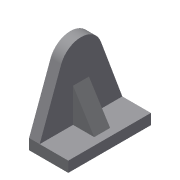
# Autodesk Inventor part: Bracket
Saved by Autodesk Inventor 2022 (Build 260148000, 148)
## iProperties
Created: 2007-03-01
Part Number: Bracket
Document SubType Name: Modeling
Designer: MFlayler
Material: Generic
Mass: 68.9563 g
Surface Area: 164.348 cm^2
Volume: 68.9563 cm^3
Density: 1 g/cm^3
Appearance: Default
Author: MFlayler
Autodesk Inventor part; units mm, degrees
ref_plane "YZ Plane" through (0, 0, 0) normal (1, 0, 0) x (0, 1, 0)
ref_plane "XZ Plane" through (0, 0, 0) normal (0, 1, 0) x (-1, 0, 0)
ref_plane "XY Plane" through (0, 0, 0) normal (0, 0, 1) x (1, 0, 0)
sketch "Sketch1" plane through (0, 0, 0) normal (0, 0, 1) x (1, 0, 0)
  line L0 (0, 54.6) -> (0, -54.6) projected
  line L1 (-7.4, 0) -> (44.4, 0) projected
  line L2 (0, -39) -> (37, -39)
  line L3 (37, -39) -> (37, 39)
  line L4 (37, 39) -> (0, 39)
  line L5 (0, 39) -> (0, -39)
  dimension "d0" = 78
  dimension "d1" = 37
  constraints: 8 end point, 2 parallel, 1 collinear, 1 horizontal, 1 perpendicular, 1 other
  measures "d0" distance of L4.end L2.start
  measures "d1" distance of L3.end L4.end
extrude "Extrusion1" add sketch "Sketch1" along normal blind 10
sketch "Sketch2" plane through (0, -39, 0) normal (-1, 0, 0) x (0, 0, 1)
  line L0 (10, 0) -> (10, 78) projected
  line L1 (0, 0) -> (10, 0) projected
  arc A0 (64.9146, 20.2333) -> (64.9146, 57.7667) centre (58, 39) ccw
  line L2 (10, 78) -> (64.9146, 57.7667)
  line L3 (10, 0) -> (64.9146, 20.2333)
  line L4 (10, 39) -> (96.3921, 39) construction
  dimension "d4" = 20
  dimension "d5" = 48
  constraints: 6 end point, 2 point on circle, 2 tangent, 1 centre point, 1 midpoint, 1 parallel, 1 point on line
  measures "d4" radius of A0
  measures "d5" distance from line of L0 A0.centre
extrude "Extrusion2" add sketch "Sketch2" against normal blind 10
sketch "Sketch4" plane through (0, 0, 0) normal (0, 1, 0) x (-1, 0, 0)
  line L0 (-37, 10) -> (-10, 10)
  line L1 (-10, 10) -> (0, 10)
  line L2 (0, 0) -> (0, 10)
  line L3 (0, 0) -> (-37, 0)
  line L4 (-37, 0) -> (-37, 10)
  line L5 (-10, 10) -> (-10, 64.9146)
  line L6 (-10, 42) -> (-30, 10)
  line L7 (-10, 42) -> (-10, 10)
  line L8 (-10, 10) -> (-30, 10)
  dimension "d12" = 32
  dimension "d13" = 20
  constraints: 18 end point, 2 collinear, 2 point on line
  measures "d12" distance of L6.start L0.end
  measures "d13" distance of L0.end L6.end
extrude "Extrusion3" add sketch "Sketch4" along normal mid plane 15 contours L6 L5 L0
body "Solid1"
